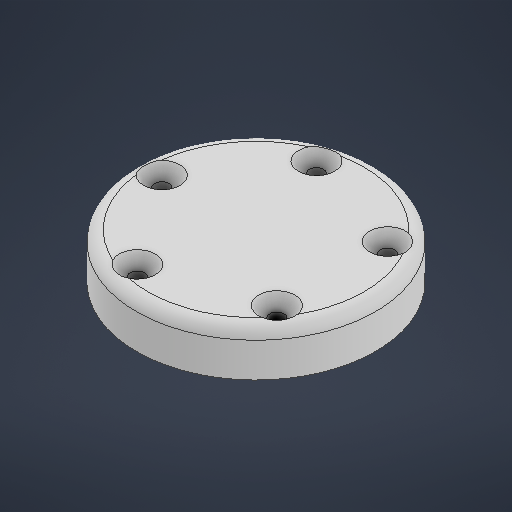
# Autodesk Inventor part: bearingplate 2
Saved by Autodesk Inventor 2026.3 (Build 303398000, 398)
## iProperties
Created: 2026-04-22
Part Number: bearingplate 2
Material: Generic
Document SubType Name: Modeling
Designer: oleg2
Density: 1 g/cm^3
Appearance: Default
Author: oleg2
Autodesk Inventor part; units mm, degrees
ref_plane "YZ Plane" through (0, 0, 0) normal (1, 0, 0) x (0, 1, 0)
ref_plane "XZ Plane" through (0, 0, 0) normal (0, 1, 0) x (-1, 0, 0)
ref_plane "XY Plane" through (0, 0, 0) normal (0, 0, 1) x (1, 0, 0)
sketch "Sketch1" plane through (0, 0, 0) normal (0, 1, 0) x (-1, 0, 0)
  circle A0 centre (0, 0) radius 33.02
  dimension "d0" = 66.04
  constraints: 1 centre point, 1 coincident
  measures "d0" diameter of A0
extrude "Extrusion1" add sketch "Sketch1" along normal blind 12.7
fillet "Fillet1" radius 3.175 1 edges at (33.02, 12.7, 0)
sketch "Sketch2" plane through (0, 12.7, 0) normal (0, 1, 0) x (1, 0, 0)
  line L0 (0, 0) -> (-26.035, 0)
  point P0 (-8.0453, -24.7608)
  point P1 (21.0628, -15.303)
  point P2 (21.0628, 15.303)
  point P3 (-8.0453, 24.7608)
  dimension "d4" = 26.035
  dimension "d7" = 360
  constraints: 2 end point, 1 coincident, 1 horizontal, 6 other
  measures "d4" distance of L0.start L0.end
hole "Hole1" at (-26.035, 12.7, 0) at (-8.0453, 12.7, 24.7608) at (21.0628, 12.7, 15.303) at (21.0628, 12.7, -15.303) at (-8.0453, 12.7, -24.7608) direction (0, -1, 0) diameter 4 end through all countersink diameter 10 countersink angle 90
sketch "Sketch3" plane through (0, 0, 0) normal (0, -1, 0) x (1, 0, 0)
  circle A0 centre (0, 0) radius 22.225
  dimension "d16" = 44.45
  constraints: 1 centre point, 1 coincident
  measures "d16" diameter of A0
extrude "Extrusion2" cut sketch "Sketch3" against normal blind 6.35
chamfer "Chamfer1" distance 6.35 angle 45 1 edges at (-22.225, 6.35, 0)
body "Solid1"
